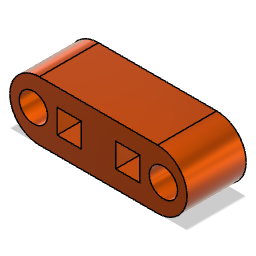
Braço robótico 3.0 (Ante-braço) v10 (Autodesk Fusion 360 design; units mm, degrees)
Autodesk Fusion 360 part; units mm, degrees
sketch "Sketch2" plane through (0, 0, 0) normal (0, 1, 0) x (1, 0, 0)
  line L0 (0, 0) -> (150, 0)
  line L1 (150, 0) -> (150, 50)
  line L2 (150, 50) -> (0, 50)
  line L3 (0, 50) -> (0, 0)
  dimension "d11" = 150
  dimension "d12" = 50
  constraint horizontal L0
  constraint vertical L1
  constraint horizontal L2
  constraint vertical L3
  constraint coincident L0.start L3.end
  measures "d11" distance of L0.start L0.end
  measures "d12" distance of L0.start L2.end
extrude "Extrude2" add sketch "Sketch2" along normal blind 50
fillet "Fillet3" radius 25 4 edges at (0, 50, -25) (0, 0, -25) (150, 50, -25) (150, 0, -25)
sketch "Sketch3" plane through (0, 0, 0) normal (0, 0, 1) x (1, 0, 0)
  arc A0 (125, 0) -> (125, 50) centre (125, 25) ccw
  line L0 (125, 50) -> (25, 50)
  arc A1 (25, 50) -> (25, 0) centre (25, 25) ccw
  line L1 (25, 0) -> (125, 0)
  circle A2 centre (20, 25) radius 12
  circle A3 centre (130, 25) radius 12
  dimension "d19" = 24
  dimension "d20" = 24
  measures "d19" diameter of A2
  measures "d20" diameter of A3
extrude "Extrude3" cut sketch "Sketch3" against normal blind 105 contours A2 | A3
sketch "Sketch4" plane through (0, 0, 0) normal (0, 0, 1) x (1, 0, 0)
  line L0 (110.0001, 14.8) -> (89.6001, 14.8)
  line L1 (89.6001, 14.8) -> (89.6001, 35.2)
  line L2 (89.6001, 35.2) -> (110.0001, 35.2)
  line L3 (110.0001, 35.2) -> (110.0001, 14.8)
  line L4 (40, 35.2) -> (60.4, 35.2)
  line L5 (60.4, 35.2) -> (60.4, 14.8)
  line L6 (60.4, 14.8) -> (40, 14.8)
  line L7 (40, 14.8) -> (40, 35.2)
  constraint horizontal L0
  constraint vertical L1
  constraint horizontal L2
  constraint vertical L3
  constraint horizontal L4
  constraint vertical L5
  constraint horizontal L6
  constraint vertical L7
extrude "Extrude4" cut sketch "Sketch4" against normal blind 25
sketch "Sketch5" plane through (0, 0, 0) normal (0, 0, 1) x (1, 0, 0)
  line L0 (60.4, 35.2) -> (60.4, 14.8)
  line L1 (60.4, 14.8) -> (40, 14.8)
  line L2 (40, 14.8) -> (40, 35.2)
  line L3 (40, 35.2) -> (60.4, 35.2)
  line L4 (89.6001, 14.8) -> (89.6001, 35.2)
  line L5 (89.6001, 35.2) -> (110.0001, 35.2)
  line L6 (110.0001, 35.2) -> (110.0001, 14.8)
  line L7 (110.0001, 14.8) -> (89.6001, 14.8)
  circle A0 centre (20, 25) radius 12
  circle A1 centre (130, 25) radius 12
  arc A2 (125, 0) -> (125, 50) centre (125, 25) ccw
  line L8 (125, 50) -> (25, 50)
  arc A3 (25, 50) -> (25, 0) centre (25, 25) ccw
  line L9 (25, 0) -> (125, 0)
  circle A4 centre (50.2, 25) radius 2.5
  circle A5 centre (99.8001, 25) radius 2.5
  dimension "d39" = 5
  dimension "d40" = 5
  measures "d39" diameter of A4
  measures "d40" diameter of A5
extrude "Extrude5" cut sketch "Sketch5" against normal blind 85 contours A4 | A5
sketch "Sketch6" plane through (0, 0, 0) normal (0, 0, 1) x (1, 0, 0)
  circle A0 centre (50.2, 25) radius 8
  circle A1 centre (99.8, 25) radius 8
  dimension "d43" = 16
  dimension "d44" = 16
  measures "d43" diameter of A0
  measures "d44" diameter of A1
extrude "Extrude6" cut sketch "Sketch6" against normal blind 26
sketch "Sketch7" plane through (0, 0, 0) normal (0, 0, 1) x (1, 0, 0)
  line L0 (60.4, 35.2) -> (60.4, 14.8)
  line L1 (60.4, 14.8) -> (40, 14.8)
  line L2 (40, 14.8) -> (40, 35.2)
  line L3 (40, 35.2) -> (60.4, 35.2)
  line L4 (89.6001, 14.8) -> (89.6001, 35.2)
  line L5 (89.6001, 35.2) -> (110.0001, 35.2)
  line L6 (110.0001, 35.2) -> (110.0001, 14.8)
  line L7 (110.0001, 14.8) -> (89.6001, 14.8)
  circle A0 centre (20, 25) radius 12
  circle A1 centre (130, 25) radius 12
  arc A2 (125, 0) -> (125, 50) centre (125, 25) ccw
  line L8 (125, 50) -> (25, 50)
  arc A3 (25, 50) -> (25, 0) centre (25, 25) ccw
  line L9 (25, 0) -> (125, 0)
  circle A4 centre (42.1991, 33.0009) radius 1.1
  circle A5 centre (58.2009, 33.0009) radius 1.1
  circle A6 centre (58.2009, 16.9991) radius 1.1
  circle A7 centre (42.1991, 16.9991) radius 1.1
  circle A8 centre (91.7992, 33.001) radius 1.1
  circle A9 centre (91.7992, 16.999) radius 1.1
  circle A10 centre (107.801, 16.9992) radius 1.1
  circle A11 centre (107.801, 33.0008) radius 1.1
  dimension "d48" = 2.2
  dimension "d49" = 2.2
  dimension "d50" = 2.2
  dimension "d51" = 2.2
  dimension "d53" = 2.2
  dimension "d54" = 2.2
  dimension "d55" = 2.2
  dimension "d56" = 2.2
  measures "d48" diameter of A4
  measures "d49" diameter of A5
  measures "d50" diameter of A6
  measures "d51" diameter of A7
  measures "d53" diameter of A8
  measures "d54" diameter of A9
  measures "d55" diameter of A10
  measures "d56" diameter of A11
sketch "Sketch8" plane through (0, 0, -50) normal (0, 0, -1) x (-1, 0, 0)
  circle A0 centre (-50.2, 25) radius 2.5
  circle A1 centre (-99.8001, 25) radius 2.5
  circle A2 centre (-20, 25) radius 12
  circle A3 centre (-130, 25) radius 12
  arc A4 (-125, 50) -> (-125, 0) centre (-125, 25) ccw
  line L0 (-125, 0) -> (-25, 0)
  arc A5 (-25, 0) -> (-25, 50) centre (-25, 25) ccw
  line L1 (-25, 50) -> (-125, 50)
  line L2 (-107.801, 16.9992) -> (-105.9894, 15.4871)
  line L3 (-110.0001, 35.2, -25) -> (-110.0001, 14.8, -25)
  line L4 (-107.801, 33.0008, 0) -> (-110.0001, 29.3796, -25)
  line L5 (-89.6001, 14.8, -25) -> (-89.6001, 35.2, -25)
  line L6 (-91.7992, 33.001, 0) -> (-89.6001, 28.0451, -25)
  line L7 (-91.7992, 16.999) -> (-88.5659, 15.2744)
  line L8 (-58.2009, 33.0009) -> (-55, 31)
  line L9 (-42.1991, 33.0009) -> (-38, 28)
  line L10 (-58.2009, 16.9991) -> (-57, 14)
  line L11 (-42.1991, 16.9991) -> (-41, 14)
  dimension "d60" = 6.53
  measures "d60" distance of L9.start L9.end
hole "Hole1" at (107.801, 33.0008, -50) at (91.7992, 33.001, -50) at (91.7992, 16.999, -50) at (107.801, 16.9992, -50) at (58.2009, 16.9991, -50) at (58.2009, 33.0009, -50) at (42.1991, 33.0009, -50) at (42.1991, 16.9991, -50) direction (0, 0, 1) diameter 1.775 depth 35 tip angle 118 counterbore diameter 4 counterbore depth 2
thread "Thread1" "ISO Metric profile 2.2 M2.2x0.45 6H"
